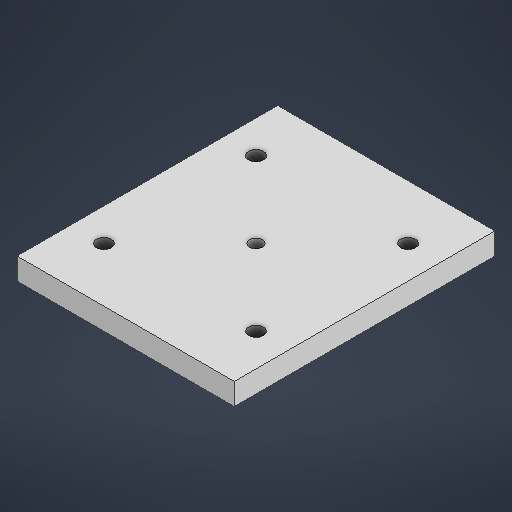
# Autodesk Inventor part: Bottom link plate
Saved by Autodesk Inventor 2026.3 (Build 303398000, 398)
## iProperties
Created: 2026-07-28
Part Number: Bottom link plate
Material: Generic
Document SubType Name: Sheet Metal
Designer: matot
Density: 1 g/cm^3
Sheet Metal Rule: Default_mm
Appearance: Default
Author: matot
Autodesk Inventor part; units mm, degrees
ref_plane "YZ Plane" through (0, 0, 0) normal (1, 0, 0) x (0, 1, 0)
ref_plane "XZ Plane" through (0, 0, 0) normal (0, 1, 0) x (-1, 0, 0)
ref_plane "XY Plane" through (0, 0, 0) normal (0, 0, 1) x (1, 0, 0)
sketch "Sketch1" plane through (0, 0, 0) normal (0, 1, 0) x (-1, 0, 0)
  line L0 (0, 0) -> (-50, 0)
  line L1 (-50, 0) -> (-50, -60)
  line L2 (-50, -60) -> (0, -60)
  line L3 (0, -60) -> (0, 0)
  point P0 (-7.5, -12.5)
  point P1 (-7.5, -47.5)
  point P2 (-42.5, -47.5)
  point P3 (-42.5, -12.5)
  dimension "d0" = 60
  dimension "d1" = 50
  dimension "d2" = 35
  dimension "d3" = 12.5
  dimension "d4" = 35
  dimension "d5" = 35
  dimension "d6" = 7.5
  dimension "d7" = 7.5
  dimension "d23" = 35
  dimension "d24" = 12.5
  constraints: 8 end point, 2 parallel, 1 horizontal, 1 perpendicular
  measures "d0" distance of L2.end L0.start
  measures "d1" distance of L1.end L2.end
  measures "d2" distance of point (-7.5, -47.5) point (-7.5, -12.5)
  measures "d3" distance from line of L0 point (-7.5, -12.5)
  measures "d4" distance of point (-42.5, -12.5) point (-7.5, -12.5)
  measures "d5" distance of point (-42.5, -47.5) point (-7.5, -47.5)
  measures "d6" distance from line of point (-7.5, -47.5) L3
  measures "d7" distance from line of L3 point (-7.5, -12.5)
  measures "d23" distance of point (-42.5, -47.5) point (-42.5, -12.5)
  measures "d24" distance from line of L0 point (-42.5, -12.5)
extrude "Extrusion1" add sketch "Sketch1" along normal blind 5
sketch "Sketch2" plane through (0, 5, 0) normal (0, 1, 0) x (1, 0, 0)
  line L0 (50, 60) -> (0, 60) projected
  line L1 (0, 60) -> (0, 0) projected
  point P0 (7.5, 12.5)
  point P1 (7.5, 47.5)
  point P2 (42.5, 47.5)
  point P3 (42.5, 12.5)
  dimension "d10" = 35
  dimension "d11" = 35
  dimension "d12" = 35
  dimension "d13" = 12.5
  dimension "d14" = 7.5
  dimension "d15" = 7.5
  dimension "d25" = 35
  dimension "d26" = 12.5
  measures "d10" distance of point (7.5, 47.5) point (7.5, 12.5)
  measures "d11" distance of point (42.5, 47.5) point (7.5, 47.5)
  measures "d12" distance of point (42.5, 12.5) point (7.5, 12.5)
  measures "d13" distance from line of L0 point (7.5, 47.5)
  measures "d14" distance from line of L1 point (7.5, 47.5)
  measures "d15" distance from line of L1 point (7.5, 12.5)
  measures "d25" distance of point (42.5, 12.5) point (42.5, 47.5)
  measures "d26" distance from line of L0 point (42.5, 47.5)
hole "Hole1" at (7.5, 5, -12.5) at (7.5, 5, -47.5) at (42.5, 5, -47.5) at (42.5, 5, -12.5) direction (0, -1, 0) diameter 3.4587 end through all thread size "M4x0.5" class "6H" standard "ISO Metric profile"
sketch "Sketch3" plane through (0, 5, 0) normal (0, 1, 0) x (1, 0, 0)
  line L0 (0, 0) -> (50, 0) projected
  line L1 (0, 60) -> (0, 0) projected
  point P0 (25, 30)
  dimension "d27" = 30
  dimension "d28" = 25
  measures "d27" distance from line of point (25, 30) L0
  measures "d28" distance from line of L1 point (25, 30)
hole "Hole2" at (25, 5, -30) direction (0, -1, 0) diameter 3 end through all
equation "\"d21\" = Thickness"
equation "\"BendRadius\" = Thickness"
equation "\"BendReliefWidth\" = Thickness"
equation "\"BendReliefDepth\" = 0.5 * Thickness"
equation "\"CornerReliefSize\" = 4 * Thickness"
equation "\"MinimumRemnant\" = 2 * Thickness"
equation "\"TransitionRadius\" = BendRadius"
equation "\"JacobiRadiusSize\" = BendRadius"
equation "\"GapSize\" = Thickness"
equation "\"Thickness\" = 0.5"
body "Solid1"
